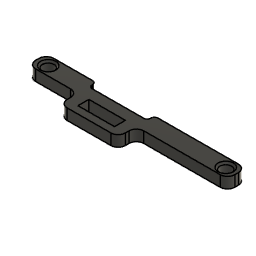
c9000c04-ed2d-4394-954b-89a0cc4c2beb (Autodesk Fusion 360 design; units mm, degrees)
Autodesk Fusion 360 part; units mm, degrees
sketch "Esboço1" plane through (0, 0, 4) normal (0, 0, 1) x (-0.999992, -0.004045, 0)
  arc A0 (-23.3506, 25.8488) -> (-21.3425, 27.8406) centre (-23.3425, 27.8487) ccw
  line L0 (-21.3425, 27.8406) -> (-21.3066, 36.725)
  arc A1 (-27.3167, 34.2406) -> (-21.3066, 36.725) centre (-25.5, 38.3576) ccw
  line L1 (-27.3167, 34.2406) -> (-27.3425, 27.8649)
  arc A2 (-27.3425, 27.8649) -> (-25.3506, 25.8568) centre (-25.3425, 27.8568) ccw
  line L2 (-25.3506, 25.8568) -> (-23.3506, 25.8488)
  circle A3 centre (-24.3405, 28.3528) radius 1.5
  circle A4 centre (-24.3405, 28.3528) radius 1.6
  circle A5 centre (24.2677, 28.3615) radius 1.6
  circle A6 centre (24.2677, 28.3615) radius 1.5
  line L3 (-24.3405, 28.3528) -> (24.2677, 28.3615) construction
  line L4 (27.2636, 27.8571) -> (27.2636, 28.8571)
  line L5 (-27.3364, 28.8571) -> (-27.3364, 27.8571)
  line L6 (-27.3364, 25.8571) -> (27.2636, 30.8571) construction
  line L7 (27.2636, 25.8571) -> (-27.3364, 30.8571) construction
  arc A7 (25.2636, 25.8571) -> (27.2636, 27.8571) centre (25.2636, 27.8571) ccw
  arc A8 (27.2636, 28.8571) -> (25.2636, 30.8571) centre (25.2636, 28.8571) ccw
  arc A9 (-25.3364, 30.8571) -> (-27.3364, 28.8571) centre (-25.3364, 28.8571) ccw
  arc A10 (-27.3364, 27.8571) -> (-25.3364, 25.8571) centre (-25.3364, 27.8571) ccw
  line L8 (0.6636, 30.8571) -> (10.6636, 30.8571)
  line L9 (10.6636, 30.8571) -> (10.6636, 33.8571)
  line L10 (10.6636, 33.8571) -> (0.6636, 33.8571)
  line L11 (0.6636, 33.8571) -> (0.6636, 30.8571)
  line L12 (11.6636, 35.8571) -> (-0.3364, 35.8571)
  line L13 (-1.4364, 27.8571) -> (12.7636, 27.8571)
  line L14 (13.6636, 32.8571) -> (13.6636, 33.8571)
  line L15 (13.6636, 26.9571) -> (13.6636, 26.7571)
  line L16 (-2.3364, 26.9571) -> (-2.3364, 26.7571)
  line L17 (-25.3364, 25.8571) -> (-3.2364, 25.8571)
  line L18 (14.5636, 25.8571) -> (25.2636, 25.8571)
  arc A11 (13.6636, 26.7571) -> (14.5636, 25.8571) centre (14.5636, 26.7571) ccw
  line L19 (-2.3364, 33.8571) -> (-2.3364, 32.8571)
  line L20 (-2.3364, 28.5678) -> (-2.3364, 27.8571)
  line L21 (25.2636, 30.8571) -> (15.6636, 30.8571)
  line L22 (10.6636, 30.8571) -> (0.6636, 30.8571)
  line L23 (-4.3364, 30.8571) -> (-25.3364, 30.8571)
  arc A12 (13.6636, 32.8571) -> (15.6636, 30.8571) centre (15.6636, 32.8571) ccw
  arc A13 (13.6636, 33.8571) -> (11.6636, 35.8571) centre (11.6636, 33.8571) ccw
  arc A14 (-0.3364, 35.8571) -> (-2.3364, 33.8571) centre (-0.3364, 33.8571) ccw
  arc A15 (-4.3364, 30.8571) -> (-2.3364, 32.8571) centre (-4.3364, 32.8571) ccw
  arc A16 (13.6636, 26.9571) -> (12.7636, 27.8571) centre (12.7636, 26.9571) ccw
  arc A17 (-1.4364, 27.8571) -> (-2.3364, 26.9571) centre (-1.4364, 26.9571) ccw
  arc A18 (-3.2364, 25.8571) -> (-2.3364, 26.7571) centre (-3.2364, 26.7571) ccw
  point P0 (-0.0364, 28.3571)
  dimension "d623" = 3.2
  dimension "d624" = 3.2
  dimension "d627" = 2
  dimension "d628" = 5
  dimension "d629" = 54.6
  dimension "d630" = 3
  dimension "d631" = 10
  dimension "d633" = 28
  dimension "d635" = 5
  dimension "d637" = 2
  dimension "d640" = 0.9
  constraint concentric A3 A4
  constraint concentric A5 A6
  constraint coincident A3.centre A4.centre
  constraint coincident A5.centre A6.centre
  constraint horizontal L17
  constraint perpendicular L4 L17
  constraint parallel L17 L21
  constraint parallel L4 L5
  constraint coincident L6 P0
  constraint coincident L7 P0
  constraint midpoint L3 P0
  constraint coincident L7.start L4
  constraint coincident L7.start L17
  constraint tangent L4 A7
  constraint tangent A7 L17
  constraint coincident L6.end L4
  constraint coincident L6.end L21
  constraint tangent L4 A8
  constraint tangent A8 L21
  constraint equal A7 A8
  constraint coincident L7.end L21
  constraint coincident L7.end L5
  constraint tangent A9 L21
  constraint tangent L5 A9
  constraint equal A7 A9
  constraint coincident L6.start L5
  constraint coincident L6.start L17
  constraint tangent L5 A10
  constraint tangent A10 L17
  constraint equal A7 A10
  constraint horizontal L8
  constraint vertical L9
  constraint horizontal L10
  constraint vertical L11
  constraint perpendicular L15 L17
  constraint perpendicular L16 L17
  constraint collinear L17 L18
  constraint tangent L18 A11
  constraint tangent L15 A11
  constraint coincident L7 L20.start
  constraint collinear L19 L20
  constraint collinear L21 L22
  constraint collinear L22 L23
  constraint tangent L21 A12
  constraint tangent L14 A12
  constraint tangent L14 A13
  constraint tangent L12 A13
  constraint equal A12 A13
  constraint tangent L12 A14
  constraint tangent L19 A14
  constraint equal A12 A14
  constraint tangent L19 A15
  constraint tangent L23 A15
  constraint equal A12 A15
  constraint tangent L15 A16
  constraint tangent L13 A16
  constraint coincident L20.end L13
  constraint coincident L20.end L16
  constraint tangent L13 A17
  constraint tangent L16 A17
  constraint tangent L16 A18
  constraint tangent L17 A18
  constraint equal A17 A18
  constraint equal A16 A18
  constraint equal A11 A18
  measures "d623" diameter of A4
  measures "d624" diameter of A5
  measures "d627" radius of A7
  measures "d628" distance of L17 L21
  measures "d629" distance of L4 L5
  measures "d630" distance of L8.start L10.end
  measures "d631" distance of L9.end L10.end
  measures "d633" distance of L5 L11
  measures "d635" distance of L8 L17
  measures "d637" radius of A12
  measures "d640" radius of A18
extrude "Extrusão1" add sketch "Esboço1" along normal blind 3 contours A0 L0 L2 L5 A9 A10 L17 L23 | A0 L0 L4 A7 A8 L12 L13 L14 L15 L16 L17 L18 A11 L19 L21 L23 A12 A13 A14 A15 A16 A17 A18
chamfer "Chanfro1" distance 0.5 angle 45 2 edges at (25.949, -28.8266, 7) (-22.6587, -29.032, 7)
